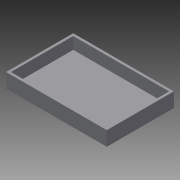
# Autodesk Inventor part: travel base
Saved by Autodesk Inventor 2015 (Build 190159000, 159)
## iProperties
Created: 2015-01-07
Part Number: travel base
Material: Generic
Document SubType Name: Modeling
Designer: harrykuperstein
Density: 1 g/cm^3
Appearance: Default
Author: harrykuperstein
Autodesk Inventor part; units mm, degrees
ref_plane "YZ Plane" through (0, 0, 0) normal (1, 0, 0) x (0, 1, 0)
ref_plane "XZ Plane" through (0, 0, 0) normal (0, 1, 0) x (-1, 0, 0)
ref_plane "XY Plane" through (0, 0, 0) normal (0, 0, 1) x (1, 0, 0)
sketch "Sketch1" plane through (0, 0, 0) normal (0, 1, 0) x (-1, 0, 0)
  line L0 (0, 0) -> (0, 711.2)
  line L1 (0, 711.2) -> (1066.8, 711.2)
  line L2 (0, 0) -> (1066.8, 0)
  line L3 (1066.8, 711.2) -> (1066.8, 0)
  dimension "d0" = 711.2
  dimension "d1" = 1066.8
  constraints: 8 end point, 2 horizontal, 1 perpendicular, 1 vertical
  measures "d0" distance of L0.start L0.end
  measures "d1" distance of L0.end L1.end
extrude "Extrusion1" add sketch "Sketch1" along normal blind 152.4
shell "Shell1" thickness 25.4 removed faces 1 at (-355.6, 152.4, 474.1333)
body "Solid1"
